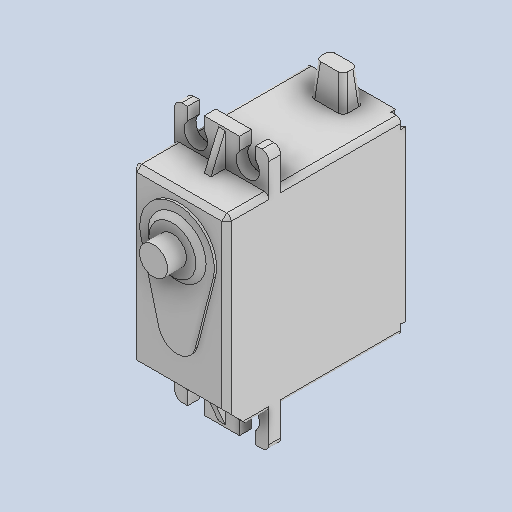
# Autodesk Inventor part: DatanS1213AnalogFeedback
Saved by Autodesk Inventor 2025.2 (Build 292293000, 293)
## iProperties
Created: 2025-02-09
Part Number: DatanS1213AnalogFeedback
Material: Generic
Document SubType Name: Modeling
Designer: LattePanda
Density: 1 g/cm^3
Appearance: Default
Author: LattePanda
Autodesk Inventor part; units mm, degrees
ref_plane "YZ Plane" through (0, 0, 0) normal (1, 0, 0) x (0, 1, 0)
ref_plane "XZ Plane" through (0, 0, 0) normal (0, 1, 0) x (-1, 0, 0)
sketch "Sketch1" plane through (0, 0, 0) normal (0, 0, 1) x (1, 0, 0)
  line L0 (-10, -20) -> (10, -20)
  line L1 (10, -20) -> (10, 20)
  line L2 (10, 20) -> (-10, 20)
  line L3 (-10, 20) -> (-10, -20)
  line L4 (-10, -20) -> (10, 20) construction
  line L5 (10, -20) -> (-10, 20) construction
  point P0 (0, 0)
  dimension "d0" = 40
  dimension "d1" = 20
  constraints: 12 end point, 2 midpoint, 2 parallel, 1 horizontal, 1 perpendicular
  measures "d0" distance of L0.end L1.end
  measures "d1" distance of L1.end L2.end
extrude "Extrusion1" add sketch "Sketch1" against normal blind 38
fillet "Fillet2" radius 1 4 edges at (-10, 20, -19) (10, 20, -19) (-10, -20, -19) (10, -20, -19)
ref_plane "Work Plane1" through (0, 0, -9) normal (0, 0, 1) x (1, 0, 0)
sketch "Sketch2" plane through (0, 0, -9) normal (0, 0, 1) x (1, 0, 0)
  line L0 (10, -19) -> (-10, -19)
  line L1 (-10, -19) -> (-10, -27.5)
  line L2 (-10, -27.5) -> (10, -27.5)
  line L3 (10, -27.5) -> (10, -19)
  line L4 (-10, 19) -> (-10, -19) projected
  line L5 (-9, -20) -> (9, -20) projected
  line L6 (10, 19) -> (10, -19) projected
  line L7 (10, 0) -> (-10, 0)
  line L8 (10, 19) -> (-10, 19)
  line L9 (-10, 19) -> (-10, 27.5)
  line L10 (-10, 27.5) -> (10, 27.5)
  line L11 (10, 27.5) -> (10, 19)
  line L12 (10, -23) -> (-10, -23) construction
  line L13 (0, -27.5) -> (0, -20) construction
  circle A0 centre (5.5, -23) radius 2.5
  line L14 (8, -20.5) -> (3, -20.5) construction
  line L15 (3, -20.5) -> (3, -25.5) construction
  line L16 (3, -25.5) -> (8, -25.5) construction
  line L17 (8, -25.5) -> (8, -20.5) construction
  line L18 (8, -20.5) -> (3, -25.5) construction
  line L19 (3, -20.5) -> (8, -25.5) construction
  line L20 (7.25, -27.5) -> (3.75, -27.5)
  line L21 (3.75, -27.5) -> (3.75, -24.7854)
  line L22 (3.75, -24.7854) -> (7.25, -24.7854)
  line L23 (7.25, -24.7854) -> (7.25, -27.5)
  line L24 (5.5, -24.7854) -> (5.5, -23) construction
  circle A1 centre (-5.5, -23) radius 2.5
  line L25 (-3.75, -27.5) -> (-3.75, -24.7854)
  line L26 (-7.25, -24.7854) -> (-7.25, -27.5)
  circle A2 centre (5.5, 23) radius 2.5
  line L27 (3.75, 27.5) -> (3.75, 24.7854)
  line L28 (7.25, 24.7854) -> (7.25, 27.5)
  line L29 (-7.25, 24.7854) -> (-7.25, 27.5)
  line L30 (-3.75, 27.5) -> (-3.75, 24.7854)
  circle A3 centre (-5.5, 23) radius 2.5
  point P0 (0, 0)
  dimension "d8" = 5
  dimension "d7" = 7.5
  dimension "d9" = 2
  dimension "d10" = 2
  dimension "d11" = 3.5
  constraints: 56 end point, 18 symmetric about line, 7 horizontal, 7 midpoint, 6 parallel, 4 point on line, 4 vertical, 3 perpendicular, 1 collinear, 12 other
  measures "d7" distance between parallel lines of L2 L5
  measures "d9" distance between parallel lines of L3 L17
  measures "d10" distance between parallel lines of L2 L16
  measures "d11" distance of L20.end L20.start
extrude "Extrusion2" add sketch "Sketch2" against normal blind 2.5 contours L3 L2 L23 A0 L21 L25 A1 L26 L1 L0 | L8 L9 L10 L29 A3 L30 L27 A2 L28 L11
fillet "Fillet3" radius 1.5 4 edges at (-10, 27.5, -10.25) (10, 27.5, -10.25) (-10, -27.5, -10.25) (10, -27.5, -10.25)
sketch "Sketch3" plane through (0, 0, -38) normal (0, 0, -1) x (-1, 0, 0)
  arc A0 (-10, -19) -> (-9, -20) centre (-9, -19) ccw projected
  line L0 (-9, -20) -> (9, -20) projected
  arc A1 (9, -20) -> (10, -19) centre (9, -19) ccw projected
  line L1 (10, -19) -> (10, 19) projected
  arc A2 (10, 19) -> (9, 20) centre (9, 19) ccw projected
  line L2 (9, 20) -> (-9, 20) projected
  arc A3 (-9, 20) -> (-10, 19) centre (-9, 19) ccw projected
  line L3 (-10, 19) -> (-10, -19) projected
  circle A4 centre (9, 19) radius 1.5
  circle A5 centre (-9, 19) radius 1.5
  circle A6 centre (9, -19) radius 1.5
  circle A7 centre (-9, -19) radius 1.5
  point P0 (0, 0)
  dimension "d15" = 3
  constraints: 4 centre point, 4 coincident, 3 equal radius
  measures "d15" diameter of A4
extrude "Extrusion3" cut sketch "Sketch3" against normal blind 1 contours L3 A7 L0 A0 | A0 L0 A7 L3 | A5 L2 A3 L3 | L3 A3 L2 A5 | A6 L1 A1 L0 | L0 A1 L1 A6 | A4 L1 A2 L2 | L2 A2 L1 A4
sketch "Sketch4" plane through (10, -19, 0) normal (1, 0, 0) x (0, 0, -1)
  line L0 (9, 0) -> (9, -7) projected
  line L1 (9, 39) -> (9, 38) projected
  line L2 (9, 0) -> (9, 38) construction
  line L3 (9, -1) -> (0, -1) projected
  line L4 (4.5, -1) -> (0, 3.5)
  line L5 (0, 0) -> (0, 38) projected
  line L6 (0, -1) -> (0, 0) projected
  point P0 (0, 19)
  dimension "d18" = 4.5
  dimension "d19" = 4.5
  constraints: 4 end point, 1 midpoint, 1 point on line, 1 vertical
  measures "d18" distance from line of L0 L4.start
  measures "d19" distance from line of L4.end L3
extrude "Extrusion4" cut sketch "Sketch4" against normal through all
sketch "Sketch5" plane through (0, 0, 0) normal (0, 0, 1) x (1, 0, 0)
  circle A0 centre (0, 10) radius 7.9
  line L0 (10, -15.5) -> (10, 19) projected
  line L1 (-10, 19) -> (-10, -15.5) projected
  line L2 (9, 20) -> (-9, 20) projected
  line L3 (0, 17.9) -> (0, -5.6)
  circle A1 centre (0, -5.6) radius 4
  line L4 (7.6491, 8.025) -> (3.873, -6.6)
  line L5 (-7.6491, 8.025) -> (-3.873, -6.6)
  point P0 (0, 0)
  dimension "d22" = 15.8
  dimension "d23" = 10
  dimension "d24" = 10
  dimension "d25" = 10
  dimension "d26" = 23.5
  dimension "d27" = 8
  constraints: 6 end point, 5 point on circle, 4 tangent, 2 centre point, 1 coincident, 1 point on line, 1 vertical
  measures "d22" diameter of A0
  measures "d23" distance from line of L0 A0.centre
  measures "d24" distance from line of L1 A0.centre
  measures "d25" distance from line of L2 A0.centre
  measures "d26" distance of L3.start L3.end
  measures "d27" diameter of A1
extrude "Extrusion5" add sketch "Sketch5" along normal blind 0.5
sketch "Sketch6" plane through (0, 0, 0.5) normal (0, 0, 1) x (1, 0, 0)
  arc A0 (7.6491, 8.025) -> (-7.6491, 8.025) centre (0, 10) ccw projected
  circle A1 centre (0, 10) radius 6.17
  point P0 (0, 0)
  dimension "d30" = 12.34
  constraints: 1 centre point, 1 coincident
  measures "d30" diameter of A1
extrude "Extrusion6" add sketch "Sketch6" along normal blind 1 draft -50
sketch "Sketch7" plane through (0, 10, 1.5) normal (0, 0, 1) x (1, 0, 0)
  circle A0 centre (0, 0) radius 4.9782 projected
  circle A1 centre (0, 0) radius 3
  point P0 (0, -10)
  dimension "d33" = 6
  constraints: 1 centre point, 1 coincident
  measures "d33" diameter of A1
extrude "Extrusion7" add sketch "Sketch7" along normal blind 4 contours A1
sketch "Sketch8" plane through (0, 0, 0) normal (1, 0, 0) x (0, 1, 0)
  line L0 (-24.7854, -9) -> (-27.5, -9) projected
  line L1 (-27, -9) -> (-20, -6)
  line L2 (-20, -9) -> (-20, -4.5) projected
  line L3 (-20, -9) -> (-20, -6)
  line L4 (-20, -9) -> (-27, -9)
  point P0 (0, 0)
  dimension "d36" = 3
  dimension "d37" = 7
  constraints: 6 end point, 2 point on line, 1 collinear, 1 horizontal
  measures "d36" distance of L2.start L1.end
  measures "d37" horizontal distance of L1.start L1.end
extrude "Extrusion8" add sketch "Sketch8" along normal mid plane 1.4
mirror "Mirror1" about plane through (0, 0, 0) normal (0, 1, 0) of "Extrusion8"
sketch "Sketch9" plane through (-9, 20, -11.5) normal (0, 1, 0) x (1, 0, 0)
  line L0 (5.25, 0) -> (12.75, 0) projected
  line L1 (9, 0) -> (9, 26.5) construction
  line L2 (1.118, 26.5) -> (16.882, 26.5) projected
  line L3 (12.5, 19.7) -> (5.5, 19.7)
  line L4 (5.5, 19.7) -> (5.5, 24)
  line L5 (5.5, 24) -> (12.5, 24)
  line L6 (12.5, 24) -> (12.5, 19.7)
  line L7 (12.5, 19.7) -> (5.5, 24) construction
  line L8 (5.5, 19.7) -> (12.5, 24) construction
  point P0 (9, -11.5)
  point P1 (9, 21.85)
  dimension "d40" = 2.5
  dimension "d41" = 7
  dimension "d42" = 4.3
  constraints: 14 end point, 4 midpoint, 2 parallel, 1 horizontal, 1 perpendicular, 1 point on line
  measures "d40" distance between parallel lines of L2 L5
  measures "d41" distance of L4.end L5.end
  measures "d42" distance between parallel lines of L3 L5
extrude "Extrusion9" add sketch "Sketch9" along normal blind 7 draft -5
fillet "Fillet4" radius 1 4 edges at (3.1938, 23.5, -31.5062) (3.1938, 23.5, -35.1938) (-3.1938, 23.5, -31.5062) (-3.1938, 23.5, -35.1938)
chamfer "Chamfer1" distance 1 angle 45 5 edges at (0, 20, 0) (-9.7071, 19.7071, 0) (-10, 1.75, 0) (9.7071, 19.7071, 0) (10, 1.75, 0)
equation "\"d10\" = d9"
equation "\"d19\" = d18"
equation "\"d24\" = d23"
equation "\"d25\" = d23"
body "Solid1"
